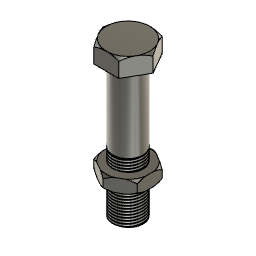
gyakorlati 7 csavar (Autodesk Fusion 360 design; units mm, degrees)
Autodesk Fusion 360 part; units mm, degrees
note: some values were not read from the file. Chosen so that the rebuilt part matches the saved one: which face or edge a step refers to.
sketch "Sketch1" plane through (0, 0, 0) normal (0, 0, 1) x (1, 0, 0)
  line L0 (50, 28.8675) -> (0, 57.735)
  line L1 (0, 57.735) -> (-50, 28.8675)
  line L2 (-50, 28.8675) -> (-50, -28.8675)
  line L3 (-50, -28.8675) -> (0, -57.735)
  line L4 (0, -57.735) -> (50, -28.8675)
  line L5 (50, -28.8675) -> (50, 28.8675)
  circle A0 centre (0, 0) radius 45
  circle A1 centre (0, 0) radius 35
  constraint coincident A0.centre A1.centre
extrude "Extrude1" add sketch "Sketch1" along normal blind 30 contours A0 makes body 1
extrude "Extrude2" add sketch "Sketch1" along normal blind 30 contours L0 L1 L2 L3 L4 L5 bodies 1
sketch "Sketch1 (2)" plane through (0, 0, 60) normal (0, 0, 1) x (-1, 0, 0) in component "teteje"
  circle A0 centre (0, 0) radius 35
  circle A1 centre (0, 0) radius 35
  constraint concentric A0 A1
extrude "Extrude1'" add sketch "Sketch1 (2)" along normal blind 175 separate body makes body 2 in component "teteje"
sketch "Sketch3" plane through (0, 0, 235) normal (0, 0, 1) x (-1, 0, 0)
  circle A0 centre (0, 0) radius 35
  circle A1 centre (0, 0) radius 35
  line L0 (-28.8675, 50) -> (-57.735, 0)
  line L1 (-57.735, 0) -> (-28.8675, -50)
  line L2 (-28.8675, -50) -> (28.8675, -50)
  line L3 (28.8675, -50) -> (57.735, 0)
  line L4 (57.735, 0) -> (28.8675, 50)
  line L5 (28.8675, 50) -> (-28.8675, 50)
  constraint coincident A0.centre A1.centre
extrude "Extrude2'" add sketch "Sketch3" along normal blind 40 contours A0 A1 | L0 L1 L2 L3 L4 L5 bodies 2 in component "teteje"
sketch "Sketch4" plane through (0, 0, 0) normal (1, 0, 0) x (0, 1, 0)
sketch "Sketch5" plane through (0, 0, 0) normal (1, 0, 0) x (0, 1, 0)
  line L0 (61, 30) -> (69, 30)
  line L1 (69, 30) -> (69, 20)
  line L2 (69, 20) -> (61, 30)
  line L3 (74, 275) -> (61, 275)
  line L4 (61, 275) -> (74, 259.381)
  line L5 (74, 259.381) -> (74, 275)
  line L6 (-62, 30) -> (-62, 20)
  line L7 (-62, 20) -> (-51, 30)
  line L8 (-51, 30) -> (-62, 30)
  constraint horizontal L0
  constraint perpendicular L0 L1
  constraint horizontal L3
  constraint perpendicular L3 L5
  constraint vertical L6
  constraint perpendicular L6 L8
revolve "Revolve1" cut sketch "Sketch5" angle 360 about axis through (0, 0, 0) along (0, 0, -1) contours L6 L7 L8 bodies 1
sketch "Sketch6" plane through (0, 0, 0) normal (1, 0, 0) x (0, 1, 0)
  line L0 (-62, 0) -> (-51, 0)
  line L1 (-51, 0) -> (-62, 10)
  line L2 (-62, 10) -> (-62, 0)
  constraint horizontal L0
  constraint perpendicular L0 L2
revolve "Revolve2" cut sketch "Sketch6" angle 360 about axis through (0, 0, 0) along (0, 0, -1) bodies 1
extrude "Extrude4" add sketch "Sketch1" along normal blind 60 and the other way blind 80 contours A1 bodies 1
thread "Thread3" "ISO Metric profile 70.0 M70x6 6g" major diameter 69.62 minor diameter 62.7358 pitch 6 angle 60 modelled right hand crest width 0.8424 on face at (34.9565, -1.7446, -53.3333) crest through (34.81, 0, -81.5) on face at (34.8261, -3.4849, 50) crest through (34.81, 0, 28.5) on bodies 1
sketch "Sketch7" plane through (0, 0, 0) normal (1, 0, 0) x (0, 1, 0)
sketch "Sketch8" plane through (0, 0, 0) normal (0, 1, 0) x (1, 0, 0)
  line L0 (-70, -275) -> (-70, -260)
  line L1 (-70, -260) -> (-50, -275)
  line L2 (-50, -275) -> (-70, -275)
  constraint vertical L0
  constraint perpendicular L0 L2
sketch "Sketch9" plane through (0, 0, 275) normal (0, 0, 1) x (-1, 0, 0)
  line L0 (28.8675, 50) -> (-28.8675, 50)
  line L1 (-28.8675, 50) -> (-57.735, 0)
  line L2 (-57.735, 0) -> (-28.8675, -50)
  line L3 (-28.8675, -50) -> (28.8675, -50)
  line L4 (28.8675, -50) -> (57.735, 0)
  line L5 (57.735, 0) -> (28.8675, 50)
  circle A0 centre (0, 0) radius 35.1683
  constraint coincident A0.centre origin
extrude "Extrude3" cut sketch "Sketch9" against normal blind 25 contours A0 bodies 2 in component "teteje"
revolve "Revolve1'" cut sketch "Sketch8" angle 360 about axis through (0, 0, 275) along (0, 0, 1) bodies 2 in component "teteje"
extrude "Extrude4'" add 1 faces at (-6.9192, -3.9627, 250) along direction (0, 0, 1) blind 25 on bodies 2 bodies 2 in component "teteje"
component "teteje" placed x (1, 0, 0) y (0, 1, 0) z (0, 0, 1) at (0, 0, 0)
